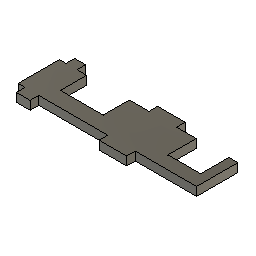
5thLessonPartDesign v2 (Autodesk Fusion 360 design; units mm, degrees)
Autodesk Fusion 360 part; units mm, degrees
sketch "Sketch1" plane through (0, 0, 0) normal (0, 0, 1) x (1, 0, 0)
  line L0 (-15, 10) -> (-15, 22)
  line L1 (-15, 22) -> (-13.1, 22)
  line L2 (-13.1, 22) -> (-13.1, 24.5)
  line L3 (-13.1, 24.5) -> (-9.9, 24.5)
  line L4 (-9.9, 24.5) -> (-9.9, 22)
  line L5 (-9.9, 22) -> (-7.1, 22)
  line L6 (-7.1, 22) -> (-7.1, 14.4)
  line L7 (-7.1, 14.4) -> (5.3, 14.4)
  line L8 (5.3, 14.4) -> (5.3, 22)
  line L9 (5.3, 22) -> (11, 22)
  line L10 (11, 22) -> (11, 24.5)
  line L11 (11, 24.5) -> (19, 24.5)
  line L12 (19, 24.5) -> (19, 22)
  line L13 (19, 22) -> (24.7, 22)
  line L14 (34.2, 22) -> (36.8, 22)
  line L15 (36.8, 22) -> (36.8, 10)
  line L16 (36.8, 10) -> (19, 10)
  line L17 (19, 10) -> (19, 7.5)
  line L18 (19, 7.5) -> (11, 7.5)
  line L19 (11, 7.5) -> (11, 10)
  line L20 (11, 10) -> (-9, 10)
  line L21 (-9, 10) -> (-9, 7.5)
  line L22 (-9, 7.5) -> (-13, 7.5)
  line L23 (-13, 7.5) -> (-13, 10)
  line L24 (-13, 10) -> (-15, 10)
  line L25 (24.7, 22) -> (24.7, 13.8)
  line L26 (34.2, 22) -> (34.2, 13.8)
  line L27 (24.7, 13.8) -> (34.2, 13.8)
  dimension "d1" = 12
  dimension "d2" = 1.9
  dimension "d3" = 2.5
  dimension "d4" = 3.2
  dimension "d5" = 2.5
  dimension "d6" = 2.8
  dimension "d7" = 7.6
  dimension "d8" = 12.4
  dimension "d9" = 7.6
  dimension "d10" = 5.7
  dimension "d11" = 2.5
  dimension "d12" = 8
  dimension "d13" = 2.5
  dimension "d14" = 5.7
  dimension "d18" = 2.6
  dimension "d19" = 12
  dimension "d20" = 17.8
  dimension "d21" = 2.5
  dimension "d22" = 8
  dimension "d23" = 2.5
  dimension "d24" = 20
  dimension "d25" = 2.5
  dimension "d26" = 4
  dimension "d27" = 2.5
  dimension "d28" = 8.2
  dimension "d29" = 8.2
  constraint vertical L0
  constraint horizontal L1
  constraint perpendicular L1 L2
  constraint perpendicular L2 L3
  constraint perpendicular L3 L4
  constraint perpendicular L4 L5
  constraint perpendicular L5 L6
  constraint perpendicular L6 L7
  constraint perpendicular L7 L8
  constraint perpendicular L8 L9
  constraint perpendicular L9 L10
  constraint perpendicular L10 L11
  constraint perpendicular L11 L12
  constraint perpendicular L12 L13
  constraint perpendicular L14 L15
  constraint perpendicular L15 L16
  constraint perpendicular L16 L17
  constraint perpendicular L17 L18
  constraint perpendicular L18 L19
  constraint perpendicular L19 L20
  constraint perpendicular L20 L21
  constraint perpendicular L21 L22
  constraint perpendicular L22 L23
  constraint perpendicular L13 L25
  constraint perpendicular L14 L26
  constraint perpendicular L26 L27
  measures "d1" distance of L0.start L0.end
  measures "d2" distance of L0.end L1.end
  measures "d3" distance of L1.end L2.end
  measures "d4" distance of L2.end L3.end
  measures "d5" distance of L3.end L4.end
  measures "d6" distance of L4.end L5.end
  measures "d7" distance of L5.end L6.end
  measures "d8" distance of L6.end L7.end
  measures "d9" distance of L7.end L8.end
  measures "d10" distance of L8.end L9.end
  measures "d11" distance of L9.end L10.end
  measures "d12" distance of L10.end L11.end
  measures "d13" distance of L11.end L12.end
  measures "d14" distance of L12.end L13.end
  measures "d18" distance of L14.start L14.end
  measures "d19" distance of L14.end L15.end
  measures "d20" distance of L15.end L16.end
  measures "d21" distance of L16.end L17.end
  measures "d22" distance of L17.end L18.end
  measures "d23" distance of L18.end L19.end
  measures "d24" distance of L19.end L20.end
  measures "d25" distance of L20.end L21.end
  measures "d26" distance of L21.end L22.end
  measures "d27" distance of L22.end L23.end
  measures "d28" distance of L13.end L25.end
  measures "d29" distance of L14.start L26.end
extrude "Extrude1" add sketch "Sketch1" along normal blind 2.5
